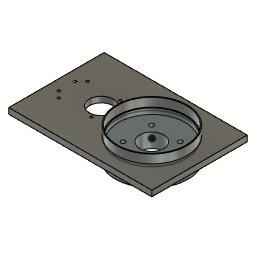
motor_holder v3 (Autodesk Fusion 360 design; units mm, degrees)
Autodesk Fusion 360 part; units mm, degrees
note: some values were not read from the file. Set by a fixed rule: which face or edge a step refers to.
sketch "Sketch1" plane through (0, 0, 0) normal (0, 0, 1) x (1, 0, 0)
  line L0 (0, 0) -> (100, 0)
  line L1 (100, 0) -> (100, 100)
  line L2 (100, 100) -> (0, 100)
  line L3 (0, 100) -> (0, 0)
  dimension "d1" = 100
  dimension "d2" = 100
  constraint horizontal L0
  constraint vertical L1
  constraint horizontal L2
  constraint vertical L3
  constraint coincident L0.start L3.end
  measures "d1" distance of L0.start L0.end
  measures "d2" distance of L0.start L2.end
extrude "Extrude1" add sketch "Sketch1" along normal blind 3 makes body 1
sketch "Sketch2" plane through (0, 0, 3) normal (0, 0, 1) x (-1, 0, 0)
  line L0 (0, -100) -> (0, 0)
  line L1 (0, 0) -> (-100, 0)
  line L2 (-100, 0) -> (-100, -100)
  line L3 (-100, -100) -> (0, -100)
  circle A0 centre (-50, -50) radius 35
  dimension "d5" = 70
  measures "d5" diameter of A0
extrude "Extrude2" cut sketch "Sketch2" against normal blind 10 contours A0 bodies 1
sketch "Sketch4" plane through (0, 0, 3) normal (0, 0, 1) x (-1, 0, 0)
  circle A0 centre (-50, -50) radius 37
  dimension "d9" = 74
  measures "d9" diameter of A0
sketch "Sketch5" plane through (0, 0, 3) normal (0, 0, 1) x (-1, 0, 0)
  circle A0 centre (-50, -50) radius 35
  line L0 (0, -100) -> (0, 0)
  line L1 (0, 0) -> (-100, 0)
  line L2 (-100, 0) -> (-100, -100)
  line L3 (-100, -100) -> (0, -100)
  circle A1 centre (-50, -50) radius 36
  dimension "d10" = 72
  constraint concentric A0 A1
  measures "d10" diameter of A1
extrude "Extrude3" add sketch "Sketch4" along normal blind 10 bodies 1
sketch "Sketch6" plane through (0, 0, 13) normal (0, 0, 1) x (-1, 0, 0)
  circle A0 centre (-50, -50) radius 37
  circle A1 centre (-50, -50) radius 36
  dimension "d13" = 72
  constraint concentric A0 A1
  measures "d13" diameter of A1
extrude "Extrude4" cut sketch "Sketch6" against normal blind 10 contours A1 bodies 1
move_face "OffsetFaces1" offset 50 1 faces at (0, 66.6667, 2) on bodies 1
sketch "Sketch7" plane through (0, 0, 0) normal (0, 0, -1) x (1, 0, 0)
  circle A0 centre (50, -50) radius 35
  line L0 (-50, 0) -> (-50, -100)
  line L1 (-50, -100) -> (100, -100)
  line L2 (100, -100) -> (100, 0)
  line L3 (100, 0) -> (-50, 0)
  line L4 (50, -50) -> (15, -50)
  line L5 (15, -50) -> (-3, -50)
  dimension "d17" = 18
  constraint coincident A0.centre L4.start
  constraint coincident A0 L4.end
  constraint horizontal L4
  constraint parallel L4 L5
  measures "d17" distance of L4.end L5.end
sketch "Sketch8" plane through (0, 0, 0) normal (0, 0, -1) x (1, 0, 0)
  circle A0 centre (-3, -50) radius 12.5
  dimension "d18" = 25
  measures "d18" diameter of A0
extrude "Extrude5" cut sketch "Sketch8" against normal blind 8 bodies 1
extrude "Extrude6" add sketch "Sketch7" along normal blind 3 bodies 1
move_body "Move1" bodies 1 to x (1, 0, 0) y (0, 1, 0) z (0, 0, 1) at (0, 0, 3)
extrude "Extrude7" cut 1 faces at (-3.7435, 53.2576, 3) along direction (0, 0, -1) blind 10 on bodies 1 bodies 1
extrude "Extrude8" cut 1 faces at (75.5273, 76.1935, 16) along direction (0, 0, -1) blind 1 on bodies 1 bodies 1
sketch "Sketch9" plane through (0, 0, 0) normal (0, 0, -1) x (1, 0, 0)
  circle A0 centre (-3, -50) radius 12.5
  circle A1 centre (50, -50) radius 35
  line L0 (100, 0) -> (-50, 0)
  line L1 (-50, 0) -> (-50, -100)
  line L2 (-50, -100) -> (100, -100)
  line L3 (100, -100) -> (100, 0)
  line L4 (-3, -50) -> (-36, -50)
  line L5 (-3, -50) -> (-3, -35)
  line L6 (-36, -50) -> (-19, -50)
  line L7 (-19, -50) -> (-19, -35)
  line L8 (-19, -35) -> (-36, -35)
  line L9 (-36, -35) -> (-36, -50)
  line L10 (-19, -50) -> (-36, -50)
  line L11 (-36, -50) -> (-36, -65)
  line L12 (-36, -65) -> (-19, -65)
  line L13 (-19, -65) -> (-19, -50)
  dimension "d27" = 33
  dimension "d28" = 15
  dimension "d29" = 17
  dimension "d30" = 15
  dimension "d31" = 17
  dimension "d32" = 15
  constraint coincident A0.centre L4.start
  constraint horizontal L4
  constraint perpendicular L4 L5
  constraint horizontal L6
  constraint vertical L7
  constraint horizontal L8
  constraint vertical L9
  constraint horizontal L10
  constraint vertical L11
  constraint horizontal L12
  constraint vertical L13
  measures "d27" distance of A0.centre L4.end
  measures "d28" distance of A0.centre L5.end
  measures "d29" distance of L4.end L6.end
  measures "d30" distance of L4.end L8.end
  measures "d31" distance of L6.end L4.end
  measures "d32" distance of L6.end L12.end
extrude "Extrude9" add sketch "Sketch9" along normal blind 2.75 contours L4 L6 L10 L11 L12 L13 | L4 L6 L7 L8 L9 L10 bodies 1
sketch "Sketch10" plane through (0, 0, 0) normal (0, 0, -1) x (1, 0, 0)
  line L0 (-19, -65) -> (-36, -65)
  line L1 (-36, -65) -> (-36, -35)
  line L2 (-36, -35) -> (-19, -35)
  line L3 (-19, -35) -> (-19, -65)
  circle A0 centre (-3, -50) radius 12.5
  circle A1 centre (50, -50) radius 35
  line L4 (100, 0) -> (-50, 0)
  line L5 (-50, 0) -> (-50, -100)
  line L6 (-50, -100) -> (100, -100)
  line L7 (100, -100) -> (100, 0)
  line L8 (-3, -50) -> (-36, -50)
  line L9 (-36, -50) -> (-36, -32.2)
  line L10 (-36, -50) -> (-36, -67.8)
  line L11 (-36, -32.2) -> (-19, -32.2)
  line L12 (-36, -67.8) -> (-19, -67.8)
  line L13 (-19, -32.2) -> (-2, -32.2)
  line L14 (-19, -67.8) -> (-2, -67.8)
  circle A2 centre (-36, -32.2) radius 1.35
  circle A3 centre (-19, -32.2) radius 1.35
  circle A4 centre (-2, -32.2) radius 1.35
  circle A5 centre (-36, -67.8) radius 1.35
  circle A6 centre (-19, -67.8) radius 1.35
  circle A7 centre (-2, -67.8) radius 1.35
  dimension "d35" = 17.8
  dimension "d36" = 17.8
  dimension "d37" = 17
  dimension "d38" = 17
  dimension "d39" = 17
  dimension "d40" = 17
  dimension "d41" = 2.7
  dimension "d42" = 2.7
  dimension "d43" = 2.7
  dimension "d44" = 2.7
  dimension "d45" = 2.7
  dimension "d46" = 2.7
  constraint coincident A0.centre L8.start
  constraint midpoint L1 L8.end
  constraint perpendicular L8 L9
  constraint perpendicular L8 L10
  constraint perpendicular L9 L11
  constraint perpendicular L10 L12
  constraint parallel L11 L13
  constraint perpendicular L1 L14
  constraint coincident L9.end L11.start
  constraint coincident L11.end L13.start
  constraint coincident L13.end A4.centre
  constraint coincident L10.end L12.start
  constraint coincident L12.end L14.start
  constraint coincident L14.end A7.centre
  measures "d35" distance of L8.end L9.end
  measures "d36" distance of L8.end L10.end
  measures "d37" distance of L9.end L11.end
  measures "d38" distance of L10.end L12.end
  measures "d39" distance of L11.end L13.end
  measures "d40" distance of L12.end L14.end
  measures "d41" diameter of A2
  measures "d42" diameter of A3
  measures "d43" diameter of A4
  measures "d44" diameter of A5
  measures "d45" diameter of A6
  measures "d46" diameter of A7
extrude "Extrude10" cut sketch "Sketch10" against normal blind 14 contours L9 L11 A2 | L9 L11 A2 | L10 L12 A5 | L10 L12 A5 | L11 L13 A3 | L11 L13 A3 | L12 L14 A6 | L12 L14 A6 | A4 | A7 bodies 1
sketch "Sketch11" plane through (0, 0, 0) normal (0, 0, -1) x (1, 0, 0)
  circle A0 centre (-19, -67.8) radius 1.35
  circle A1 centre (-36, -32.2) radius 1.35
  circle A2 centre (-2, -67.8) radius 1.35
  circle A3 centre (-36, -67.8) radius 1.35
  circle A4 centre (-19, -32.2) radius 1.35
  circle A5 centre (-2, -32.2) radius 1.35
  line L0 (-19, -65) -> (-36, -65)
  line L1 (-36, -65) -> (-36, -35)
  line L2 (-36, -35) -> (-19, -35)
  line L3 (-19, -35) -> (-19, -65)
  circle A6 centre (-3, -50) radius 12.5
  circle A7 centre (50, -50) radius 35
  line L4 (100, 0) -> (-50, 0)
  line L5 (-50, 0) -> (-50, -100)
  line L6 (-50, -100) -> (100, -100)
  line L7 (100, -100) -> (100, 0)
  line L8 (-25, -29.95) -> (15, -29.95)
  line L9 (15, -29.95) -> (15, -69.95)
  line L10 (15, -69.95) -> (-25, -69.95)
  line L11 (-25, -69.95) -> (-25, -29.95)
  dimension "d49" = 40
  dimension "d50" = 40
  constraint horizontal L8
  constraint vertical L9
  constraint horizontal L10
  constraint vertical L11
  measures "d49" distance of L8.start L8.end
  measures "d50" distance of L8.start L10.end
extrude "Extrude11" add sketch "Sketch11" along normal blind 10 separate body contours A7 makes body 2
move_face "OffsetFaces2" offset 3 1 faces at (15.0435, 48.2554, -3.3333) on bodies 2
sketch "Sketch13" plane through (0, 0, -10) normal (0, 0, -1) x (1, 0, 0)
  circle A0 centre (50, -50) radius 38
  circle A1 centre (35, -35) radius 3.25
  circle A2 centre (35, -65) radius 3.25
  circle A3 centre (65, -35) radius 3.25
  circle A4 centre (65, -65) radius 3.25
  circle A5 centre (50, -50) radius 12.5
  circle A6 centre (35, -35) radius 2.5
  circle A7 centre (65, -35) radius 2.5
  circle A8 centre (35, -65) radius 2.5
  circle A9 centre (65, -65) radius 2.5
  dimension "d69" = 30
  dimension "d70" = 30
  dimension "d71" = 30
  dimension "d72" = 6.5
  dimension "d73" = 6.5
  dimension "d74" = 6.5
  dimension "d75" = 6.5
  dimension "d76" = 25
  dimension "d77" = 5
  dimension "d78" = 5
  dimension "d79" = 5
  dimension "d80" = 5
  constraint concentric A0 A5
  constraint concentric A1 A6
  constraint concentric A3 A7
  constraint concentric A2 A8
  constraint concentric A4 A9
  measures "d69" distance of A1.centre A2.centre
  measures "d70" distance of A2.centre A4.centre
  measures "d71" distance of A3.centre A4.centre
  measures "d72" diameter of A1
  measures "d73" diameter of A2
  measures "d74" diameter of A3
  measures "d75" diameter of A4
  measures "d76" diameter of A5
  measures "d77" diameter of A6
  measures "d78" diameter of A7
  measures "d79" diameter of A8
  measures "d80" diameter of A9
extrude "Extrude13" cut sketch "Sketch13" against normal blind 10 contours A5 | A6 | A7 | A8 | A9 bodies 2
sketch "Sketch14" plane through (0, 0, -10) normal (0, 0, -1) x (1, 0, 0)
  circle A0 centre (35, -65) radius 2.5
  circle A1 centre (65, -35) radius 2.5
  circle A2 centre (65, -65) radius 2.5
  circle A3 centre (35, -35) radius 2.5
  circle A4 centre (50, -50) radius 12.5
  circle A5 centre (50, -50) radius 38
  circle A6 centre (35, -35) radius 3.25
  circle A7 centre (65, -35) radius 3.25
  circle A8 centre (35, -65) radius 3.25
  circle A9 centre (65, -65) radius 3.25
  dimension "d83" = 6.5
  dimension "d84" = 6.5
  dimension "d85" = 6.5
  dimension "d86" = 6.5
  constraint concentric A3 A6
  constraint concentric A1 A7
  constraint concentric A0 A8
  constraint concentric A2 A9
  measures "d83" diameter of A6
  measures "d84" diameter of A7
  measures "d85" diameter of A8
  measures "d86" diameter of A9
extrude "Extrude14" cut sketch "Sketch14" against normal blind 4 contours A6 | A7 | A8 | A9 bodies 2
extrude "Extrude15" add 1 faces at (44.5362, 72.5231, -10) along direction (0, 0, -1) blind 5 on bodies 2 bodies 2
sketch "Sketch15" plane through (0, 0, 0) normal (0, 0, -1) x (1, 0, 0)
  circle A0 centre (-19, -67.8) radius 1.35
  circle A1 centre (-36, -32.2) radius 1.35
  circle A2 centre (-2, -67.8) radius 1.35
  circle A3 centre (-36, -67.8) radius 1.35
  circle A4 centre (-19, -32.2) radius 1.35
  circle A5 centre (-2, -32.2) radius 1.35
  line L0 (-19, -65) -> (-36, -65)
  line L1 (-36, -65) -> (-36, -35)
  line L2 (-36, -35) -> (-19, -35)
  line L3 (-19, -35) -> (-19, -65)
  circle A6 centre (-3, -50) radius 12.5
  circle A7 centre (50, -50) radius 35
  line L4 (100, 0) -> (-50, 0)
  line L5 (-50, 0) -> (-50, -100)
  line L6 (-50, -100) -> (100, -100)
  line L7 (100, -100) -> (100, 0)
  line L8 (-3, -50) -> (-39, -50)
  line L9 (-39, -50) -> (-39, -41.5)
  line L10 (-39, -50) -> (-39, -58.5)
  dimension "d91" = 36
  dimension "d92" = 8.5
  dimension "d93" = 8.5
  constraint coincident A6.centre L8.start
  constraint perpendicular L3 L8
  constraint perpendicular L8 L9
  constraint perpendicular L8 L10
  measures "d91" distance of A6.centre L8.end
  measures "d92" distance of L8.end L9.end
  measures "d93" distance of L8.end L10.end
hole "Hole1" at (-39, 41.5, 0) at (-39, 58.5, 0) direction (0, 0, 1) diameter 2.7 depth 10 tip angle 118 bodies 1
move_face "OffsetFaces3" offset 2 5 faces at (-34.6768, 67.5325, 4) (-17.6567, 67.6656, 2) (-0.6917, 67.4669, 2) (-19.43, 33.4797, 2) (-35.3841, 30.9987, 2) on bodies 1
move_face "OffsetFaces4" offset 4 1 faces at (-0.6567, 32.0656, 2) on bodies 1
sketch "Sketch16" plane through (0, 0, 0) normal (0, 0, -1) x (1, 0, 0)
  circle A0 centre (-39, -41.5) radius 1.35
  circle A1 centre (-39, -58.5) radius 1.35
  line L0 (-19, -65) -> (-36, -65)
  line L1 (-36, -65) -> (-36, -35)
  line L2 (-36, -35) -> (-19, -35)
  line L3 (-19, -35) -> (-19, -65)
  circle A2 centre (-3, -50) radius 12.5
  circle A3 centre (50, -50) radius 35
  line L4 (100, 0) -> (-50, 0)
  line L5 (-50, 0) -> (-50, -100)
  line L6 (-50, -100) -> (100, -100)
  line L7 (100, -100) -> (100, 0)
  line L8 (-3, -50) -> (-3, -35)
  line L9 (-3, -50) -> (-3, -65)
  line L10 (-3, -35) -> (2, -35)
  line L11 (-3, -65) -> (2, -65)
  line L12 (2, -35) -> (-14.5, -35)
  line L13 (2, -35) -> (-32.5, -35)
  line L14 (-3, -65) -> (-19.5, -65)
  line L15 (2, -65) -> (-32.5, -65)
  dimension "d99" = 15
  dimension "d100" = 15
  dimension "d101" = 5
  dimension "d102" = 5
  dimension "d103" = 16.5
  dimension "d104" = 34.5
  dimension "d105" = 16.5
  dimension "d106" = 34.5
  constraint coincident A2.centre L8.start
  constraint perpendicular L4 L8
  constraint parallel L8 L9
  constraint perpendicular L8 L10
  constraint perpendicular L9 L11
  constraint perpendicular L3 L12
  constraint parallel L12 L13
  constraint perpendicular L9 L14
  constraint parallel L0 L15
  measures "d99" distance of A2.centre L8.end
  measures "d100" distance of A2.centre L9.end
  measures "d101" distance of L8.end L10.end
  measures "d102" distance of L9.end L11.end
  measures "d103" distance of L10.end L12.end
  measures "d104" distance of L10.end L13.end
  measures "d105" distance of L9.end L14.end
  measures "d106" distance of L11.end L15.end
move_face "OffsetFaces5" offset -3 1 faces at (-30.3333, 65, -1.8333) on bodies 1
move_face "OffsetFaces6" offset -3 1 faces at (-24.6667, 35, -0.9167) on bodies 1
hole "Hole2" at (-32.5, 35, 0) at (-32.5, 65, 0) at (2, 35, 0) at (2, 65, 0) direction (0, 0, 1) diameter 2.7 depth 10 tip angle 118 bodies 1
extrude "Extrude16" cut 1 faces at (-30.3333, 54, -2.75) along direction (0, 0, 1) blind 1 on bodies 1 bodies 1
move_face "OffsetFaces7" offset 0.2 4 faces at (67.4969, 65.1246, -2) (67.4876, 35.2489, -4) (37.4876, 35.2489, -4) (32.6508, 65.8551, -2) on bodies 2
equation "d35 = ( 35.6 / 2 ) * 1 mm"
equation "d36 = ( 35.6 / 2 ) * 1 mm"
equation "d92 = ( 17 / 2 ) * 1 mm"
equation "d93 = ( 17 / 2 ) * 1 mm"
